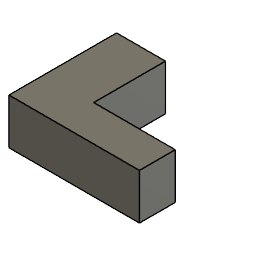
replay (Autodesk Fusion 360 design; units mm, degrees)
Autodesk Fusion 360 part; units mm, degrees
ref_plane "工作平面1" through (0, 17, 0) normal (0, 1, 0) x (0, 0, 1)
sketch "草图1" plane through (0, 17, 0) normal (0, 1, 0) x (1, 0, 0)
  line L0 (9, -5) -> (9, -27)
  line L1 (9, -27) -> (34, -27)
  line L2 (34, -27) -> (34, -38)
  line L3 (34, -38) -> (-6, -38)
  line L4 (-6, -38) -> (-6, -5)
  line L5 (-6, -5) -> (9, -5)
extrude "拉伸1" add sketch "草图1" against normal blind 14
